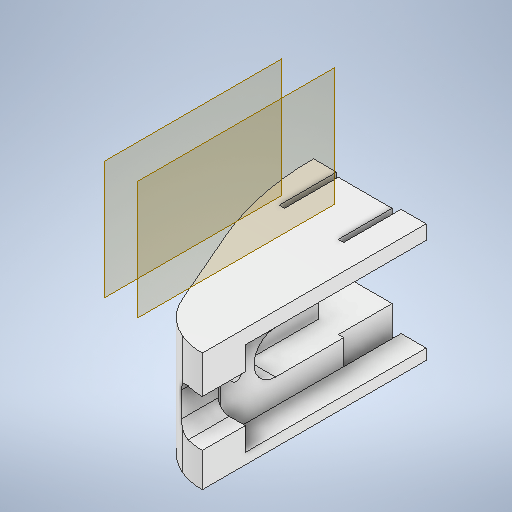
# Autodesk Inventor part: MontageAufnahmeLO-LH
Saved by Autodesk Inventor 2025 (Build 290162010, 162A)
## iProperties
Created: 2024-11-18
Part Number: MontageAufnahmeLO-LH
Material: PC/ABS-Kunststoff, 3DDruck, PLA
Document SubType Name: Modeling
Designer: Admin
Density: 1.1 g/cm^3
Appearance: Glatt - Weiß(2)
Mass: 29.2248 g
Surface Area: 64.7654 cm^2
Volume: 26.568 cm^3
Author: Admin
Autodesk Inventor part; units mm, degrees
ref_plane "YZ Plane" through (0, 0, 0) normal (1, 0, 0) x (0, 1, 0)
ref_plane "XZ Plane" through (0, 0, 0) normal (0, 1, 0) x (-1, 0, 0)
ref_plane "XY Plane" through (0, 0, 0) normal (0, 0, 1) x (1, 0, 0)
sketch "Skizze1" plane through (0, 0, 0) normal (0, 0, 1) x (1, 0, 0)
  line L0 (-9, -921.9811) -> (9, -921.9811)
  arc A0 (0.1765, -974.1575) -> (9, -982.9811) centre (15.7474, -967.4101) ccw
  line L1 (0.1765, -974.1575) -> (9, -974.1575) construction
  line L2 (9, -982.9811) -> (9, -974.1575)
  line L3 (9, -982.9811) -> (4, -982.9811) construction
  line L4 (9, -937.9811) -> (9, -974.1575)
  line L5 (-9, -952.9811) -> (0.1765, -974.1575)
  line L6 (7.5, -920.9811) -> (-7.5, -920.9811) projected
  line L7 (-7.5, -920.9811) -> (-7.5, -905.9811) projected
  line L8 (-7.5, -905.9811) -> (-9, -905.9811) projected
  line L9 (-9, -905.9811) -> (-9, -937.9811) projected
  line L10 (-9, -937.9811) -> (-7.5, -937.9811) projected
  line L11 (-7.5, -937.9811) -> (-7.5, -922.9811) projected
  line L12 (-7.5, -922.9811) -> (7.5, -922.9811) projected
  line L13 (7.5, -922.9811) -> (7.5, -937.9811) projected
  line L14 (7.5, -937.9811) -> (9, -937.9811) projected
  line L15 (9, -937.9811) -> (9, -905.9811) projected
  line L16 (9, -905.9811) -> (7.5, -905.9811) projected
  line L17 (7.5, -905.9811) -> (7.5, -920.9811) projected
  line L18 (-9, -937.9811) -> (-9, -952.9811)
  arc A1 (-15.4279, -921.9811) -> (-9, -952.9811) centre (62.5385, -921.9811) ccw
  line L19 (-15.4279, -921.9811) -> (-9, -921.9811)
  line L20 (-9, -921.9811) -> (-9, -937.9811)
  arc A2 (9, -982.9811) -> (16, -984.4325) centre (16, -966.8272) ccw
  line L21 (16, -984.4325) -> (16, -921.9811)
  line L22 (16, -921.9811) -> (9, -921.9811)
  line L23 (-9.05, -948.4314) -> (0.95, -948.4314)
  line L24 (-9.05, -935.8314) -> (-9.05, -948.4314)
  line L25 (0.95, -948.4314) -> (0.95, -935.8314)
  line L26 (0.95, -935.8314) -> (-9.05, -935.8314)
  line L27 (16, -972.4325) -> (9, -972.4325)
  line L28 (9, -972.4325) -> (8.5, -972.4325)
  line L29 (8.5, -972.4325) -> (8.5, -982.7547)
  point P0 (0, 0)
  dimension "d0" = 5
  dimension "d1" = 45
  dimension "d4" = 15
  dimension "d56" = 7
  dimension "d61" = 12
  dimension "d65" = 0.5
  constraints: 36 end point, 7 perpendicular, 7 point on circle, 5 vertical, 4 horizontal, 3 centre point, 3 point on line, 3 tangent, 2 line through centre, 2 midpoint, 1 coincident, 1 collinear, 4 other
  measures "d0" distance of L3.start L3.end
  measures "d1" distance of L4.start L3.start
  measures "d4" distance of L9.end L5.start
  measures "d56" distance between parallel lines of L21 L4
  measures "d61" distance from line of L27 L21.start
  measures "d65" distance of L27.end L28.end
extrude "Extrusion1" add sketch "Skizze1" against normal blind 30 contours L9 L26 L24 L23 L18 A1 L19 | L9 L18 L23 L24 L26 | L4 L28 L29 A0 L5 L18 L23 L25 L26 L11 L12 L13 L14 | L10 L11 L26 L25 L23 L18
sketch "Skizze3" plane through (0, 0, 0) normal (0, 0, 1) x (1, 0, 0)
  circle A0 centre (-13.05, -942.1314) radius 1.621 construction
  line L0 (-13.05, -942.1314) -> (-6.55, -942.1314) construction
  line L1 (-6.55, -942.1314) -> (-1.55, -942.1314) construction
  point P0 (0, 0)
  dimension "d14" = 6.5
  dimension "d15" = 5
  constraints: 4 coincident, 4 end point, 1 horizontal, 1 point on line
  measures "d14" distance of L0.start L0.end
  measures "d15" distance of L0.end L1.end
hole "Bohrung2" at (-6.55, -942.1314, 0) at (-1.55, -942.1314, 0) direction (0, 0, -1) diameter 1.567 depth 10 tip angle 118 thread size "M2x0.4" class "6H" standard "ANSI Metric M Profile"
sketch "Skizze7" plane through (-7.5, -937.9811, 0) normal (-1, 0, 0) x (0, 0, 1)
  line L0 (0, 15) -> (-30, 15) projected
  line L1 (-9, 15) -> (-21, 15)
  line L2 (-21, 15) -> (-21, 1)
  line L3 (-9, 1) -> (-9, 15)
  line L4 (-15, 15) -> (-15, 1)
  line L5 (-21, 1) -> (-15, 1)
  line L6 (-9, 1) -> (-15, 1)
  point P0 (0, 937.9811)
  point P1 (-9, 8)
  point P2 (-21, 15)
  dimension "d40" = 14
  dimension "d41" = 12
  constraints: 12 end point, 3 midpoint, 2 equal length, 2 horizontal, 1 collinear, 1 perpendicular, 1 point on line
  measures "d40" distance of L4.start L4.end
  measures "d41" distance from line of point (-9, 8) L2
extrude "Extrusion2" cut sketch "Skizze7" against normal through all
ref_plane "Arbeitsebene1" through (-1, -982.9811, 0) normal (1, 0, 0) x (0, 0, -1)
sketch "Skizze5" plane through (-1, -982.9811, 0) normal (1, 0, 0) x (0, 0, -1)
  line L0 (30, 45) -> (30, 10.5485) projected
  point P0 (0, 982.9811)
  point P1 (15, 15)
  point P2 (30, 0)
  dimension "d31" = 15
  dimension "d32" = 15
  measures "d31" distance from line of L0 point (15, 15)
  measures "d32" horizontal distance of point (30, 0) point (15, 15)
hole "Bohrung4" at (-1, -967.9811, -15) direction (1, 0, 0) diameter 3.2 end through all start extended yes countersink diameter 6.3 countersink angle 90 clearance for "Flachkopfmaschinenschraube" size "M3" standard "ANSI Metrisches M Profil"
sketch "Skizze9" plane through (9, -982.9811, 0) normal (1, 0, 0) x (0, 0, -1)
  circle A0 centre (15, 26) radius 6
  line L0 (21, 26) -> (21, 65.5618)
  line L1 (9, 26) -> (9, 65.5618)
  line L2 (9, 65.5618) -> (21, 65.5618)
  line L3 (0, 10.5485) -> (0, 45) projected
  line L4 (30, 45) -> (30, 10.5485) projected
  line L5 (0, 61) -> (30, 61) projected
  line L6 (15, 61) -> (15, 26)
  point P0 (0, 982.9811)
  dimension "d51" = 12
  dimension "d72" = 15
  dimension "d73" = 15
  dimension "d75" = 35
  constraints: 8 end point, 3 vertical, 2 horizontal, 2 point on circle, 2 tangent, 1 centre point, 1 midpoint
  measures "d51" diameter of A0
  measures "d72" distance from line of L3 L6.end
  measures "d73" distance from line of L4 L6.end
  measures "d75" distance from line of L5 L6.end
extrude "Extrusion3" cut sketch "Skizze9" against normal blind 8
ref_plane "Arbeitsebene2" through (-10.5, -982.9811, 0) normal (1, 0, 0) x (0, 0, -1)
sketch "Skizze8" plane through (-10.5, -952.9811, 0) normal (-1, 0, 0) x (0, 0, 1)
  line L0 (-15, 7.5) -> (-15, 0)
  line L1 (0, 0) -> (-30, 0) projected
  line L2 (0, 15) -> (-30, 15) projected
  line L3 (-15, 15) -> (-15, 7.5)
  point P0 (0, 952.9811)
  point P1 (-15, 3.75)
  constraints: 4 end point, 3 midpoint, 1 collinear, 1 perpendicular, 1 vertical
hole "Bohrung5" at (-10.5, -945.4811, -15) direction (1, 0, 0) diameter 3.2 end through all start extended yes countersink diameter 6.3 countersink angle 90 clearance for "Flachkopfmaschinenschraube" size "M3" standard "ANSI Metrisches M Profil"
extrude "Extrusion4" add sketch "Skizze1" along normal blind 1 contours L0 L15 L14 L13 L12 L11 L26 L9 | L9 L26 L24 L23 L18 A1 L19 | L22 L21 L27 L4 L15 | L4 L28 L29 A0 L5 L18 L23 L25 L26 L11 L12 L13 L14 | L27 L21 A2 L2 L4 | L4 L2 A0 L29 L28
extrude "Extrusion5" add sketch "Skizze1" against normal blind 2 contours L22 L21 L27 L4 L15 | L27 L21 A2 L2 L4 | L4 L2 A0 L29 L28
extrude "Extrusion6" add sketch "Skizze1" against normal blind 8.5 contours L27 L21 A2 L2 L4 | L4 L2 A0 L29 L28
fillet "Rundung2" radius 3 1 edges at (8.5, -977.5936, -8.5)
sketch "Skizze13" plane through (0, 0, -30) normal (0, 0, -1) x (-1, 0, 0)
  arc A0 (9, -952.9811) -> (15.4279, -921.9811) centre (-62.5385, -921.9811) ccw projected
  line L0 (-0.1765, -974.1575) -> (9, -952.9811) projected
  arc A1 (-16, -984.4325) -> (-9, -982.9811) centre (-16, -966.8272) ccw projected
  arc A2 (-9, -982.9811) -> (-0.1765, -974.1575) centre (-15.7474, -967.4101) ccw projected
  line L1 (15.4279, -921.9811) -> (9, -921.9811) projected
  line L2 (9, -921.9811) -> (9, -937.9811) projected
  line L3 (9, -937.9811) -> (7.5, -937.9811) projected
  line L4 (-7.5, -922.9811) -> (-7.5, -937.9811) projected
  line L5 (7.5, -922.9811) -> (-7.5, -922.9811) projected
  line L6 (7.5, -937.9811) -> (7.5, -922.9811) projected
  line L7 (-7.5, -937.9811) -> (-9, -937.9811) projected
  line L8 (-9, -937.9811) -> (-9, -921.9811)
  line L9 (-16, -984.4325) -> (-16, -921.9811)
  line L10 (-16, -921.9811) -> (-9, -921.9811)
  line L11 (-16, -972.4325) -> (-9, -972.4325) projected
  line L12 (-8.5, -972.4325) -> (-8.5, -982.7547) projected
  line L13 (-9, -972.4325) -> (-8.5, -972.4325) projected
  point P0 (0, 0)
  constraints: 6 end point, 2 vertical, 1 collinear, 1 perpendicular
extrude "Extrusion7" add sketch "Skizze13" along normal blind 2 and the other way blind 2
extrude "Extrusion8" add sketch "Skizze13" against normal blind 8.5 contours A2 A1 L9 L11 L13 L12
fillet "Rundung3" radius 3 1 edges at (8.5, -977.5936, -21.5)
mirror "Spiegeln1" about plane through (0.2861, -953.2068, -32) normal (0, 0, -1) remove original yes
